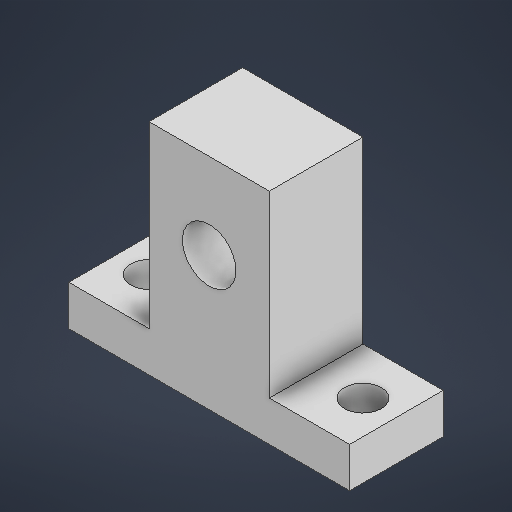
# Autodesk Inventor part: Linear Rod Holder SK8
Saved by Autodesk Inventor 2025.1 (Build 291241000, 241)
## iProperties
Created: 2024-12-18
Part Number: Linear Rod Holder SK8
Material: Generic
Document SubType Name: Modeling
Designer: jerem
Density: 1 g/cm^3
Appearance: Default
Author: jerem
Autodesk Inventor part; units mm, degrees
ref_plane "YZ Plane" through (0, 0, 0) normal (1, 0, 0) x (0, 1, 0)
ref_plane "XZ Plane" through (0, 0, 0) normal (0, 1, 0) x (-1, 0, 0)
ref_plane "XY Plane" through (0, 0, 0) normal (0, 0, 1) x (1, 0, 0)
sketch "Sketch1" plane through (0, 0, 0) normal (0, 0, 1) x (1, 0, 0)
  line L0 (21, 0) -> (-21, 0)
  line L1 (-21, 0) -> (-21, 6)
  line L2 (-9, 32.8) -> (9, 32.8)
  line L3 (21, 6) -> (21, 0)
  circle A0 centre (0, 20) radius 4
  line L4 (0, 20) -> (0, 0) construction
  line L5 (-21, 6) -> (-9, 6)
  line L6 (-9, 6) -> (-9, 32.8)
  line L7 (21, 6) -> (9, 6)
  line L8 (9, 6) -> (9, 32.8)
  dimension "d2" = 8
  dimension "d3" = 18
  dimension "d4" = 20
  dimension "d5" = 6
  dimension "d6" = 32.8
  dimension "d7" = 42
  constraints: 18 end point, 3 symmetric about line, 2 horizontal, 2 parallel, 2 perpendicular, 1 centre point, 1 midpoint, 1 vertical
  measures "d2" diameter of A0
  measures "d3" distance between parallel lines of L8 L6
  measures "d4" distance of L4.end L4.start
  measures "d5" distance between parallel lines of L0 L5
  measures "d6" distance between parallel lines of L0 L2
  measures "d7" distance between parallel lines of L3 L1
extrude "Extrusion1" add sketch "Sketch1" along normal blind 14
sketch "Sketch2" plane through (-21, 6, 0) normal (0, 1, 0) x (1, 0, 0)
  line L0 (12, 0) -> (0, 0) projected
  line L1 (0, 0) -> (0, -14) projected
  line L2 (12, -14) -> (0, -14) projected
  line L3 (12, 0) -> (12, -14) projected
  circle A0 centre (5, -7) radius 2.75
  line L4 (42, 0) -> (30, 0) projected
  line L5 (30, 0) -> (30, -14) projected
  line L6 (42, -14) -> (30, -14) projected
  line L7 (42, 0) -> (42, -14) projected
  line L8 (12, -7) -> (30, -7) construction
  line L9 (5, -7) -> (12, -7) construction
  circle A1 centre (37, -7) radius 2.75
  line L10 (37, -7) -> (30, -7) construction
  point P0 (21, 0)
  point P1 (21, -7)
  dimension "d10" = 5.5
  dimension "d11" = 16
  dimension "d12" = 5.5
  dimension "d13" = 16
  constraints: 6 end point, 3 midpoint, 2 centre point, 2 perpendicular
  measures "d10" diameter of A0
  measures "d11" distance of L9.start point (21, -7)
  measures "d12" diameter of A1
  measures "d13" distance of point (21, -7) L10.start
extrude "Extrusion2" cut sketch "Sketch2" against normal through all contours A0 | A1
equation "\"d12\" = d10"
equation "\"d13\" = d11"
body "Solid1"
